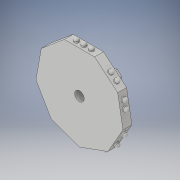
# Autodesk Inventor part: 9 ul Right Braille Wheel (Nonagon)
Saved by Autodesk Inventor 2017 (Build 210142000, 142)
## iProperties
Created: 2018-03-08
Part Number: 9 ul Right Braille Wheel (Nonagon)
Material: Generic
Document SubType Name: Modeling
Designer: Russ
Density: 1 g/cm^3
Appearance: Default
Author: Russ
Autodesk Inventor part; units mm, degrees
ref_plane "YZ Plane" through (0, 0, 0) normal (1, 0, 0) x (0, 1, 0)
ref_plane "XZ Plane" through (0, 0, 0) normal (0, 1, 0) x (-1, 0, 0)
ref_plane "XY Plane" through (0, 0, 0) normal (0, 0, 1) x (1, 0, 0)
sketch "Sketch1" plane through (0, 0, 0) normal (0, 0, 1) x (1, 0, 0)
  line L0 (0, -14.9412) -> (-9.604, -11.4456)
  line L1 (-9.604, -11.4456) -> (-14.7142, -2.5945)
  line L2 (-14.7142, -2.5945) -> (-12.9395, 7.4706)
  line L3 (-12.9395, 7.4706) -> (-5.1102, 14.0402)
  line L4 (-5.1102, 14.0402) -> (5.1102, 14.0402)
  line L5 (5.1102, 14.0402) -> (12.9395, 7.4706)
  line L6 (12.9395, 7.4706) -> (14.7142, -2.5945)
  line L7 (14.7142, -2.5945) -> (9.604, -11.4456)
  line L8 (9.604, -11.4456) -> (0, -14.9412)
  point P0 (0, 0)
  point P1 (0, 0)
  dimension "d0" = 28.9814
  constraints: 18 end point, 1 coincident, 19 other
  measures "d0" distance from line of L0.start L4
extrude "Extrusion1" add sketch "Sketch1" along normal blind 3
sketch "Sketch2" plane through (0, 0, 0) normal (0, 0, -1) x (-1, 0, 0)
  arc A0 (-2.0086, 7.3505) -> (2.0086, 7.3505) centre (0, 0) ccw
  line L0 (0, 7.62) -> (0, 9.525)
  line L1 (0, 9.525) -> (1.016, 9.525)
  line L2 (0, 9.525) -> (-1.016, 9.525)
  arc A1 (-1.4866, 7.4736) -> (1.4866, 7.4736) centre (0, 0) ccw
  line L3 (-1.4866, 7.4736) -> (-1.8582, 9.342)
  line L4 (-2.916, 7.04) -> (-3.6451, 8.8)
  line L5 (-4.2334, 6.3358) -> (-5.2918, 7.9197)
  line L6 (-5.3882, 5.3882) -> (-6.7352, 6.7352)
  line L7 (-6.3358, 4.2334) -> (-7.9197, 5.2918)
  line L8 (-7.04, 2.916) -> (-8.8, 3.6451)
  line L9 (-7.4736, 1.4866) -> (-9.342, 1.8582)
  line L10 (-7.62, 0) -> (-9.525, 0)
  line L11 (-7.4736, -1.4866) -> (-9.342, -1.8582)
  line L12 (-7.04, -2.916) -> (-8.8, -3.6451)
  line L13 (-6.3358, -4.2334) -> (-7.9197, -5.2918)
  line L14 (-5.3882, -5.3882) -> (-6.7352, -6.7352)
  line L15 (-4.2334, -6.3358) -> (-5.2918, -7.9197)
  line L16 (-2.916, -7.04) -> (-3.6451, -8.8)
  line L17 (-1.4866, -7.4736) -> (-1.8582, -9.342)
  line L18 (0, -7.62) -> (0, -9.525)
  line L19 (1.4866, -7.4736) -> (1.8582, -9.342)
  line L20 (2.916, -7.04) -> (3.6451, -8.8)
  line L21 (4.2334, -6.3358) -> (5.2918, -7.9197)
  line L22 (5.3882, -5.3882) -> (6.7352, -6.7352)
  line L23 (6.3358, -4.2334) -> (7.9197, -5.2918)
  line L24 (7.04, -2.916) -> (8.8, -3.6451)
  line L25 (7.4736, -1.4866) -> (9.342, -1.8582)
  line L26 (7.62, 0) -> (9.525, 0)
  line L27 (7.4736, 1.4866) -> (9.342, 1.8582)
  line L28 (7.04, 2.916) -> (8.8, 3.6451)
  line L29 (6.3358, 4.2334) -> (7.9197, 5.2918)
  line L30 (5.3882, 5.3882) -> (6.7352, 6.7352)
  line L31 (4.2334, 6.3358) -> (5.2918, 7.9197)
  line L32 (2.916, 7.04) -> (3.6451, 8.8)
  line L33 (1.4866, 7.4736) -> (1.8582, 9.342)
  arc A2 (-1.4866, 7.4736) -> (1.4866, 7.4736) centre (0, 0) ccw
  arc A3 (-1.016, 9.525) -> (-1.6724, 8.4079) centre (-0.1056, 8.2386) ccw
  arc A4 (1.6724, 8.4079) -> (1.016, 9.525) centre (0.1056, 8.2386) ccw
  circle A5 centre (0, 0) radius 7.62
  line L34 (-1.4866, 7.4736) -> (-1.6724, 8.4079)
  line L35 (-1.016, 9.525) -> (1.016, 9.525)
  line L36 (1.6724, 8.4079) -> (1.4866, 7.4736)
  arc A6 (-1.016, 9.525) -> (-1.6724, 8.4079) centre (-0.1056, 8.2386) ccw
  arc A7 (1.6724, 8.4079) -> (1.016, 9.525) centre (0.1056, 8.2386) ccw
  dimension "d5" = 15.24
  dimension "d6" = 360
  dimension "d7" = 1.016
  dimension "d8" = 1.016
  dimension "d9" = 1.905
  constraints: 74 end point, 14 point on circle, 7 centre point, 5 symmetric about line, 4 coincident, 3 concentric, 2 collinear, 1 perpendicular, 1 point on line, 1 vertical, 101 other
  measures "d5" diameter of A0
  measures "d7" distance of L1.start L1.end
  measures "d8" distance of L1.start L2.end
  measures "d9" distance of L0.start L1.start
extrude "Extrusion2" add sketch "Sketch2" along normal blind 3.81
pattern_circular "Circular Pattern1" count 8 over 360 about axis through (0, 0, 0) along (0, 0, -1) of "Extrusion2"
sketch "Sketch3" plane through (-5.1102, 14.0402, 0) normal (0, 1, 0) x (1, 0, 0)
  circle A0 centre (2.575, -1.5014) radius 0.8
  circle A1 centre (5.115, -1.5014) radius 0.8
  circle A2 centre (7.655, -1.5014) radius 0.8
  line L0 (-0.5079, -0.6748) -> (2.0528, -3)
  line L1 (2.0528, -3) -> (9.5277, -3)
  line L2 (9.4982, -0.3484) -> (-1.073, -0.3484)
  line L3 (-2.5018, -3) -> (9.4982, -3)
  line L4 (-2.5018, -3) -> (-1.073, -0.3484)
  line L5 (0.8768, 0) -> (0.3475, 0) projected
  line L6 (10.2204, -3) -> (0, -3) projected
  line L7 (10.2204, 0) -> (10.2204, -3) projected
  point P0 (5.1102, 0)
  point P1 (5.5277, -0.6748)
  dimension "d15" = 1.6
  dimension "d16" = 2.54
  dimension "d17" = 2.54
  dimension "d18" = 1.6
  dimension "d19" = 1.6
  dimension "d20" = 1.4605
  dimension "d21" = 1.4986
  dimension "d22" = 0
  dimension "d23" = 1.4986
  dimension "d24" = 1.4986
  dimension "d25" = 5.9944
  dimension "d27" = 0
  dimension "d28" = 5.1054
  constraints: 10 end point, 3 centre point
  measures "d15" diameter of A0
  measures "d16" distance of A1.centre A0.centre
  measures "d17" distance of A2.centre A1.centre
  measures "d18" diameter of A1
  measures "d19" diameter of A2
  measures "d20" distance from line of L0 A0.centre
  measures "d21" distance from line of L1 A2.centre
  measures "d22" distance between parallel lines of L3 L1
  measures "d23" distance from line of L1 A1.centre
  measures "d24" distance from line of L1 A0.centre
  measures "d25" distance from line of L4 A1.centre
  measures "d27" distance between parallel lines of L6 L1
  measures "d28" distance from line of L7 A1.centre
extrude "Extrusion3" add sketch "Sketch3" along normal blind 1.2
fillet "Fillet1" radius 0.8 3 edges at (1.7448, 15.2402, 1.5014) (-0.7952, 15.2402, 1.5014) (-3.3352, 15.2402, 1.5014)
sketch "Sketch4" plane through (0, 0, -3.81) normal (0, 0, -1) x (-1, 0, 0)
  circle A0 centre (0, 0) radius 1.6002
  dimension "d32" = 3.2004
  constraints: 1 centre point, 1 coincident
  measures "d32" diameter of A0
extrude "Extrusion4" cut sketch "Sketch4" against normal up to next
pattern_circular "Circular Pattern2" count 9 over 360 about axis through (0, 0, -3.81) along (0, 0, 1) of "Extrusion3"
sketch "Sketch5" plane through (0, 0, 0) normal (0, 0, -1) x (-1, 0, 0)
  line L0 (5.1102, 14.0402) -> (12.9395, 7.4706) projected
  line L1 (5.1102, 14.0402) -> (12.9395, 7.4706)
  line L2 (12.9395, 7.4706) -> (14.6272, 9.482)
  line L3 (14.6272, 9.482) -> (6.7979, 16.0515)
  line L4 (6.7979, 16.0515) -> (5.1102, 14.0402)
  line L5 (12.9395, 7.4706) -> (14.7142, -2.5945) projected
  line L6 (12.9395, 7.4706) -> (14.7142, -2.5945)
  line L7 (14.7142, -2.5945) -> (17.5585, -2.093)
  line L8 (17.5585, -2.093) -> (14.6272, 9.482)
  line L9 (-12.9395, 7.4706) -> (-5.1102, 14.0402) projected
  line L10 (-8.1123, 11.5211) -> (-9.4668, 13.1353)
  line L11 (-9.4668, 13.1353) -> (-7.1898, 15.0458)
  line L12 (-7.1898, 15.0458) -> (-5.8354, 13.4317)
  line L13 (-9.604, -11.4456) -> (-14.7142, -2.5945) projected
  line L14 (-14.7142, -2.5945) -> (-17.6536, -1.4861)
  line L15 (-17.6536, -1.4861) -> (-16.7467, 1.5365)
  line L16 (-16.7467, 1.5365) -> (-14.0691, 1.0644)
  line L17 (-14.7142, -2.5945) -> (-12.9395, 7.4706) projected
  line L18 (-12.78, -5.9446) -> (-14.6226, -7.0342)
  line L19 (-14.6226, -7.0342) -> (-13.3803, -9.1352)
  line L20 (-13.3803, -9.1352) -> (-11.45, -8.2484)
  line L21 (14.7142, -2.5945) -> (9.604, -11.4456) projected
  line L22 (12.78, -5.9446) -> (14.7387, -7.8068)
  line L23 (14.7387, -7.8068) -> (10.4839, -12.2822)
  line L24 (10.4839, -12.2822) -> (9.604, -11.4456)
  line L25 (9.604, -11.4456) -> (0, -14.9412) projected
  line L26 (0, -14.9412) -> (1.1482, -18.0959)
  line L27 (1.1482, -18.0959) -> (4.4102, -16.9086)
  line L28 (4.4102, -16.9086) -> (3.8165, -13.5521)
  line L29 (6.0711, -12.7315) -> (7.6925, -15.714)
  line L30 (7.6925, -15.714) -> (10.2125, -14.9412)
  line L31 (10.2125, -14.9412) -> (9.604, -11.4456)
  line L32 (0, -14.9412) -> (-9.604, -11.4456) projected
  line L33 (-6.0711, -12.7315) -> (-7.2039, -15.8437)
  line L34 (-7.2039, -15.8437) -> (-1.9485, -17.7565)
  line L35 (-1.9485, -17.7565) -> (-0.963, -14.5907)
  line L36 (0, -14.9412) -> (3.8165, -13.5521)
  point P0 (0, 0)
  constraints: 58 end point, 14 perpendicular, 11 point on line, 3 collinear
extrude "Extrusion5" cut sketch "Sketch5" against normal through all
fillet "Fillet2" radius 0.8 9 edges at (9.187, 12.1858, 1.5014) (11.1328, 10.5531, 1.5014) (14.4295, 5.931, 1.5014) (14.8705, 3.4295, 1.5014) (14.866, -4.7317, 1.5014) (12.326, -9.1311, 1.5014) (8.3465, -13.1804, 1.5014) (-4.4652, -14.593, 1.5014) (-14.0708, -6.109, 1.5014)
body "Solid1"
